Autodesk Fusion 360 part; units mm, degrees
(part 6 of 8)
  spline S141 degree 5 poles (61.3624, 12.8997) (61.363, 12.9) (61.3795, 12.9077) (61.4119, 12.9229) (61.4601, 12.9455) (61.524, 12.976) (61.6029, 13.0142) (61.6817, 13.0528) (61.7603, 13.092) (61.8388, 13.1316) (61.9172, 13.1716) (61.9953, 13.2121) (62.0734, 13.2531) (62.1513, 13.2945) (62.229, 13.3363) (62.3066, 13.3785) (62.3841, 13.4212) (62.4614, 13.4642) (62.5386, 13.5076) (62.6157, 13.5515) (62.6926, 13.5957) (62.7694, 13.6403) (62.846, 13.6853) (62.9225, 13.7307) (62.9989, 13.7764) (63.0751, 13.8226) (63.1512, 13.869) (63.2272, 13.9159) (63.303, 13.963) (63.3787, 14.0106) (63.4542, 14.0585) (63.5297, 14.1067) (63.605, 14.1552) (63.6801, 14.2041) (63.7552, 14.2534) (63.8301, 14.3029) (63.9049, 14.3528) (63.9795, 14.403) (64.054, 14.4536) (64.1284, 14.5044) (64.2027, 14.5556) (64.2768, 14.6071) (64.3508, 14.6589) (64.4247, 14.711) (64.4984, 14.7634) (64.572, 14.8161) (64.6455, 14.8691) (64.7189, 14.9225) (64.7921, 14.9761) (64.8652, 15.03) (64.9382, 15.0842) (65.011, 15.1387) (65.0837, 15.1935) (65.1418, 15.2375) (65.1853, 15.2707) (65.2143, 15.2928) (65.2287, 15.3039) knots 0.270845 0.270845 0.270845 0.270845 0.270845 0.270845 0.271429 0.285714 0.3 0.314286 0.328571 0.342857 0.357143 0.371429 0.385714 0.4 0.414286 0.428571 0.442857 0.457143 0.471429 0.485714 0.5 0.514286 0.528571 0.542857 0.557143 0.571429 0.585714 0.6 0.614286 0.628571 0.642857 0.657143 0.671429 0.685714 0.7 0.714286 0.728571 0.742857 0.757143 0.771429 0.785714 0.8 0.814286 0.828571 0.842857 0.857143 0.871429 0.885714 0.9 0.914286 0.928571 0.942857 0.957143 0.971429 0.985714 1 1 1 1 1 1
  arc A71 (65.2287, 15.3039) -> (64.8693, 16.7623) centre (0, 0) ccw
  spline S142 degree 5 poles (64.8693, 16.7623) (64.8513, 16.7654) (64.8153, 16.7716) (64.7614, 16.7808) (64.6895, 16.7928) (64.5997, 16.8075) (64.5099, 16.8219) (64.4201, 16.836) (64.3303, 16.8497) (64.2405, 16.8632) (64.1508, 16.8763) (64.0611, 16.8891) (63.9714, 16.9016) (63.8818, 16.9137) (63.7921, 16.9255) (63.7025, 16.937) (63.613, 16.9481) (63.5234, 16.9589) (63.4339, 16.9694) (63.3445, 16.9795) (63.255, 16.9893) (63.1656, 16.9987) (63.0763, 17.0078) (62.987, 17.0165) (62.8977, 17.0249) (62.8084, 17.0329) (62.7192, 17.0405) (62.6301, 17.0478) (62.541, 17.0547) (62.4519, 17.0612) (62.3629, 17.0674) (62.2739, 17.0732) (62.185, 17.0786) (62.0961, 17.0836) (62.0073, 17.0882) (61.9185, 17.0925) (61.8298, 17.0963) (61.7411, 17.0997) (61.6525, 17.1027) (61.564, 17.1053) (61.4755, 17.1075) (61.3871, 17.1092) (61.2987, 17.1106) (61.2105, 17.1115) (61.1223, 17.1119) (61.0341, 17.1119) (60.9461, 17.1114) (60.8581, 17.1105) (60.7702, 17.1091) (60.6824, 17.1072) (60.5947, 17.1048) (60.507, 17.1019) (60.4363, 17.0992) (60.3831, 17.0969) (60.3474, 17.0953) (60.3292, 17.0944) (60.3285, 17.0944) knots -1 -1 -1 -1 -1 -1 -0.985714 -0.971429 -0.957143 -0.942857 -0.928571 -0.914286 -0.9 -0.885714 -0.871429 -0.857143 -0.842857 -0.828571 -0.814286 -0.8 -0.785714 -0.771429 -0.757143 -0.742857 -0.728571 -0.714286 -0.7 -0.685714 -0.671429 -0.657143 -0.642857 -0.628571 -0.614286 -0.6 -0.585714 -0.571429 -0.557143 -0.542857 -0.528571 -0.514286 -0.5 -0.485714 -0.471429 -0.457143 -0.442857 -0.428571 -0.414286 -0.4 -0.385714 -0.371429 -0.357143 -0.342857 -0.328571 -0.314286 -0.3 -0.285714 -0.271429 -0.270845 -0.270845 -0.270845 -0.270845 -0.270845 -0.270845
  spline S143 degree 3 poles (60.1267, 17.239) (60.1339, 17.214) (60.1459, 17.1906) (60.1782, 17.1497) (60.1981, 17.1326) (60.2371, 17.1107) (60.2547, 17.1038) (60.2911, 17.0952) (60.3098, 17.0935) (60.3285, 17.0944) knots 0 0 0 0 0.007813 0.007813 0.015626 0.015626 0.021241 0.021241 0.026855 0.026855 0.026855 0.026855
  arc A72 (60.1267, 17.239) -> (59.7414, 18.5303) centre (0, 0) ccw
  spline S144 degree 3 poles (59.8309, 18.7618) (59.8085, 18.7486) (59.7888, 18.7312) (59.7573, 18.6897) (59.7458, 18.6661) (59.7343, 18.6228) (59.7321, 18.6041) (59.7328, 18.5667) (59.7358, 18.5481) (59.7414, 18.5303) knots 0 0 0 0 0.007813 0.007813 0.015626 0.015626 0.021241 0.021241 0.026855 0.026855 0.026855 0.026855
  spline S145 degree 5 poles (59.8309, 18.7618) (59.8315, 18.7622) (59.8472, 18.7715) (59.878, 18.7896) (59.9237, 18.8169) (59.9844, 18.8534) (60.0593, 18.899) (60.134, 18.9451) (60.2085, 18.9916) (60.2828, 19.0386) (60.3569, 19.086) (60.4308, 19.1339) (60.5045, 19.1822) (60.578, 19.2309) (60.6514, 19.28) (60.7246, 19.3295) (60.7975, 19.3794) (60.8704, 19.4297) (60.943, 19.4804) (61.0155, 19.5315) (61.0877, 19.583) (61.1598, 19.6348) (61.2318, 19.687) (61.3035, 19.7395) (61.3751, 19.7924) (61.4466, 19.8457) (61.5178, 19.8993) (61.5889, 19.9532) (61.6598, 20.0075) (61.7306, 20.0621) (61.8012, 20.117) (61.8716, 20.1723) (61.9419, 20.2279) (62.012, 20.2839) (62.0819, 20.3401) (62.1517, 20.3967) (62.2213, 20.4535) (62.2907, 20.5107) (62.36, 20.5682) (62.4292, 20.626) (62.4981, 20.6841) (62.5669, 20.7425) (62.6356, 20.8012) (62.7041, 20.8602) (62.7724, 20.9195) (62.8406, 20.9791) (62.9086, 21.0389) (62.9765, 21.0991) (63.0442, 21.1595) (63.1118, 21.2202) (63.1792, 21.2812) (63.2464, 21.3425) (63.3135, 21.404) (63.3671, 21.4535) (63.4072, 21.4907) (63.4338, 21.5155) (63.4472, 21.528) knots 0.270845 0.270845 0.270845 0.270845 0.270845 0.270845 0.271429 0.285714 0.3 0.314286 0.328571 0.342857 0.357143 0.371429 0.385714 0.4 0.414286 0.428571 0.442857 0.457143 0.471429 0.485714 0.5 0.514286 0.528571 0.542857 0.557143 0.571429 0.585714 0.6 0.614286 0.628571 0.642857 0.657143 0.671429 0.685714 0.7 0.714286 0.728571 0.742857 0.757143 0.771429 0.785714 0.8 0.814286 0.828571 0.842857 0.857143 0.871429 0.885714 0.9 0.914286 0.928571 0.942857 0.957143 0.971429 0.985714 1 1 1 1 1 1
  arc A73 (63.4472, 21.528) -> (62.9487, 22.9449) centre (0, 0) ccw
  spline S146 degree 5 poles (62.9487, 22.9449) (62.9305, 22.9462) (62.8941, 22.9489) (62.8395, 22.9528) (62.7668, 22.9578) (62.676, 22.9638) (62.5852, 22.9695) (62.4944, 22.9748) (62.4037, 22.9798) (62.3131, 22.9846) (62.2225, 22.989) (62.132, 22.993) (62.0415, 22.9968) (61.9511, 23.0002) (61.8608, 23.0033) (61.7705, 23.0061) (61.6803, 23.0085) (61.5901, 23.0106) (61.5, 23.0124) (61.41, 23.0139) (61.32, 23.015) (61.2302, 23.0157) (61.1403, 23.0161) (61.0506, 23.0162) (60.9609, 23.0159) (60.8713, 23.0152) (60.7818, 23.0142) (60.6923, 23.0129) (60.603, 23.0112) (60.5137, 23.0091) (60.4245, 23.0066) (60.3354, 23.0038) (60.2463, 23.0006) (60.1574, 22.997) (60.0685, 22.993) (59.9798, 22.9887) (59.8911, 22.9839) (59.8025, 22.9788) (59.714, 22.9732) (59.6257, 22.9672) (59.5374, 22.9609) (59.4492, 22.9541) (59.3612, 22.9469) (59.2732, 22.9392) (59.1854, 22.9312) (59.0977, 22.9227) (59.0101, 22.9137) (58.9226, 22.9043) (58.8353, 22.8944) (58.748, 22.884) (58.6609, 22.8732) (58.574, 22.8619) (58.5038, 22.8523) (58.4511, 22.8449) (58.4158, 22.8398) (58.3977, 22.8372) (58.397, 22.8371) knots -1 -1 -1 -1 -1 -1 -0.985714 -0.971429 -0.957143 -0.942857 -0.928571 -0.914286 -0.9 -0.885714 -0.871429 -0.857143 -0.842857 -0.828571 -0.814286 -0.8 -0.785714 -0.771429 -0.757143 -0.742857 -0.728571 -0.714286 -0.7 -0.685714 -0.671429 -0.657143 -0.642857 -0.628571 -0.614286 -0.6 -0.585714 -0.571429 -0.557143 -0.542857 -0.528571 -0.514286 -0.5 -0.485714 -0.471429 -0.457143 -0.442857 -0.428571 -0.414286 -0.4 -0.385714 -0.371429 -0.357143 -0.342857 -0.328571 -0.314286 -0.3 -0.285714 -0.271429 -0.270845 -0.270845 -0.270845 -0.270845 -0.270845 -0.270845
  spline S147 degree 3 poles (58.1822, 22.9616) (58.1918, 22.9374) (58.206, 22.9152) (58.242, 22.8777) (58.2636, 22.8626) (58.3045, 22.8445) (58.3226, 22.8394) (58.3597, 22.8343) (58.3785, 22.8344) (58.397, 22.8371) knots 0 0 0 0 0.007813 0.007813 0.015626 0.015626 0.021241 0.021241 0.026855 0.026855 0.026855 0.026855
  arc A74 (58.1822, 22.9616) -> (57.6741, 24.2096) centre (0, 0) ccw
  spline S148 degree 3 poles (57.7408, 24.4488) (57.7198, 24.4335) (57.7019, 24.4142) (57.6746, 24.3698) (57.6653, 24.3452) (57.6581, 24.301) (57.6576, 24.2822) (57.662, 24.2451) (57.6668, 24.2269) (57.6741, 24.2096) knots 0 0 0 0 0.007813 0.007813 0.015626 0.015626 0.021241 0.021241 0.026855 0.026855 0.026855 0.026855
  spline S149 degree 5 poles (57.7408, 24.4488) (57.7414, 24.4492) (57.7561, 24.4599) (57.785, 24.481) (57.8279, 24.5125) (57.8848, 24.5547) (57.9549, 24.6073) (58.0248, 24.6604) (58.0944, 24.7139) (58.1638, 24.7678) (58.233, 24.8222) (58.302, 24.877) (58.3707, 24.9321) (58.4392, 24.9877) (58.5075, 25.0437) (58.5755, 25.1) (58.6433, 25.1568) (58.711, 25.2139) (58.7784, 25.2713) (58.8455, 25.3292) (58.9125, 25.3874) (58.9793, 25.4459) (59.0459, 25.5048) (59.1122, 25.564) (59.1784, 25.6236) (59.2443, 25.6835) (59.3101, 25.7437) (59.3756, 25.8042) (59.441, 25.8651) (59.5061, 25.9263) (59.5711, 25.9878) (59.6359, 26.0496) (59.7004, 26.1117) (59.7648, 26.1742) (59.829, 26.2369) (59.893, 26.2999) (59.9568, 26.3633) (60.0204, 26.4269) (60.0838, 26.4908) (60.147, 26.555) (60.2101, 26.6195) (60.2729, 26.6843) (60.3356, 26.7493) (60.3981, 26.8146) (60.4604, 26.8802) (60.5225, 26.9461) (60.5844, 27.0123) (60.6462, 27.0787) (60.7077, 27.1454) (60.7691, 27.2123) (60.8303, 27.2795) (60.8913, 27.347) (60.9522, 27.4147) (61.0007, 27.4691) (61.037, 27.51) (61.0612, 27.5373) (61.0732, 27.551) knots 0.270845 0.270845 0.270845 0.270845 0.270845 0.270845 0.271429 0.285714 0.3 0.314286 0.328571 0.342857 0.357143 0.371429 0.385714 0.4 0.414286 0.428571 0.442857 0.457143 0.471429 0.485714 0.5 0.514286 0.528571 0.542857 0.557143 0.571429 0.585714 0.6 0.614286 0.628571 0.642857 0.657143 0.671429 0.685714 0.7 0.714286 0.728571 0.742857 0.757143 0.771429 0.785714 0.8 0.814286 0.828571 0.842857 0.857143 0.871429 0.885714 0.9 0.914286 0.928571 0.942857 0.957143 0.971429 0.985714 1 1 1 1 1 1
  arc A75 (61.0732, 27.551) -> (60.4403, 28.9132) centre (0, 0) ccw
  spline S150 degree 5 poles (60.4403, 28.9132) (60.422, 28.9128) (60.3856, 28.9119) (60.3309, 28.9105) (60.258, 28.9085) (60.167, 28.9057) (60.0761, 28.9026) (59.9853, 28.8991) (59.8945, 28.8954) (59.8039, 28.8913) (59.7133, 28.887) (59.6228, 28.8823) (59.5324, 28.8773) (59.4421, 28.872) (59.3519, 28.8664) (59.2617, 28.8604) (59.1717, 28.8541) (59.0818, 28.8475) (58.9919, 28.8406) (58.9022, 28.8333) (58.8125, 28.8257) (58.723, 28.8178) (58.6335, 28.8096) (58.5442, 28.801) (58.455, 28.792) (58.3659, 28.7827) (58.2768, 28.7731) (58.1879, 28.7631) (58.0992, 28.7528) (58.0105, 28.7421) (57.9219, 28.731) (57.8335, 28.7196) (57.7452, 28.7078) (57.657, 28.6957) (57.569, 28.6831) (57.481, 28.6702) (57.3932, 28.6569) (57.3056, 28.6433) (57.218, 28.6292) (57.1307, 28.6147) (57.0434, 28.5999) (56.9563, 28.5846) (56.8694, 28.5689) (56.7826, 28.5528) (56.6959, 28.5363) (56.6094, 28.5194) (56.5231, 28.502) (56.4369, 28.4842) (56.351, 28.4659) (56.2651, 28.4472) (56.1795, 28.428) (56.0941, 28.4084) (56.0252, 28.3921) (55.9734, 28.3796) (55.9387, 28.3711) (55.921, 28.3668) (55.9203, 28.3666) knots -1 -1 -1 -1 -1 -1 -0.985714 -0.971429 -0.957143 -0.942857 -0.928571 -0.914286 -0.9 -0.885714 -0.871429 -0.857143 -0.842857 -0.828571 -0.814286 -0.8 -0.785714 -0.771429 -0.757143 -0.742857 -0.728571 -0.714286 -0.7 -0.685714 -0.671429 -0.657143 -0.642857 -0.628571 -0.614286 -0.6 -0.585714 -0.571429 -0.557143 -0.542857 -0.528571 -0.514286 -0.5 -0.485714 -0.471429 -0.457143 -0.442857 -0.428571 -0.414286 -0.4 -0.385714 -0.371429 -0.357143 -0.342857 -0.328571 -0.314286 -0.3 -0.285714 -0.271429 -0.270845 -0.270845 -0.270845 -0.270845 -0.270845 -0.270845
  spline S151 degree 3 poles (55.6945, 28.4698) (55.7063, 28.4466) (55.7226, 28.426) (55.7621, 28.3921) (55.785, 28.3791) (55.8275, 28.3651) (55.846, 28.3617) (55.8834, 28.3602) (55.9021, 28.3621) (55.9203, 28.3666) knots 0 0 0 0 0.007813 0.007813 0.015626 0.015626 0.021241 0.021241 0.026855 0.026855 0.026855 0.026855
  arc A76 (55.6945, 28.4698) -> (55.0682, 29.663) centre (0, 0) ccw
  spline S152 degree 3 poles (55.1116, 29.9074) (55.0921, 29.8902) (55.0762, 29.8692) (55.0533, 29.8225) (55.0465, 29.7971) (55.0435, 29.7524) (55.0449, 29.7337) (55.0528, 29.6971) (55.0594, 29.6794) (55.0682, 29.663) knots 0 0 0 0 0.007813 0.007813 0.015626 0.015626 0.021241 0.021241 0.026855 0.026855 0.026855 0.026855
  spline S153 degree 5 poles (55.1116, 29.9074) (55.1122, 29.9079) (55.1258, 29.92) (55.1525, 29.9437) (55.1921, 29.9793) (55.2447, 30.0267) (55.3094, 30.0859) (55.3738, 30.1455) (55.438, 30.2054) (55.5019, 30.2658) (55.5655, 30.3266) (55.6288, 30.3878) (55.6919, 30.4493) (55.7547, 30.5113) (55.8173, 30.5736) (55.8795, 30.6362) (55.9416, 30.6992) (56.0034, 30.7626) (56.0649, 30.8263) (56.1262, 30.8903) (56.1873, 30.9547) (56.2481, 31.0194) (56.3087, 31.0845) (56.369, 31.1498) (56.4291, 31.2155) (56.4889, 31.2815) (56.5486, 31.3477) (56.608, 31.4143) (56.6671, 31.4812) (56.7261, 31.5484) (56.7848, 31.6159) (56.8433, 31.6837) (56.9016, 31.7518) (56.9596, 31.8201) (57.0174, 31.8888) (57.0751, 31.9577) (57.1324, 32.0269) (57.1896, 32.0963) (57.2466, 32.1661) (57.3033, 32.2361) (57.3598, 32.3063) (57.4161, 32.3769) (57.4722, 32.4477) (57.5281, 32.5187) (57.5838, 32.59) (57.6393, 32.6616) (57.6945, 32.7334) (57.7496, 32.8055) (57.8044, 32.8778) (57.859, 32.9503) (57.9135, 33.0231) (57.9677, 33.0962) (58.0217, 33.1695) (58.0648, 33.2283) (58.097, 33.2725) (58.1184, 33.302) (58.1291, 33.3168) knots 0.270845 0.270845 0.270845 0.270845 0.270845 0.270845 0.271429 0.285714 0.3 0.314286 0.328571 0.342857 0.357143 0.371429 0.385714 0.4 0.414286 0.428571 0.442857 0.457143 0.471429 0.485714 0.5 0.514286 0.528571 0.542857 0.557143 0.571429 0.585714 0.6 0.614286 0.628571 0.642857 0.657143 0.671429 0.685714 0.7 0.714286 0.728571 0.742857 0.757143 0.771429 0.785714 0.8 0.814286 0.828571 0.842857 0.857143 0.871429 0.885714 0.9 0.914286 0.928571 0.942857 0.957143 0.971429 0.985714 1 1 1 1 1 1
  arc A77 (58.1291, 33.3168) -> (57.3676, 34.6115) centre (0, 0) ccw
  spline S154 degree 5 poles (57.3676, 34.6115) (57.3495, 34.6094) (57.3133, 34.605) (57.259, 34.5983) (57.1866, 34.5893) (57.0963, 34.5777) (57.0062, 34.5658) (56.9161, 34.5536) (56.8261, 34.5411) (56.7363, 34.5284) (56.6465, 34.5153) (56.5569, 34.5019) (56.4674, 34.4882) (56.378, 34.4742) (56.2888, 34.4599) (56.1996, 34.4453) (56.1106, 34.4303) (56.0217, 34.4151) (55.933, 34.3995) (55.8444, 34.3836) (55.7559, 34.3674) (55.6675, 34.3509) (55.5793, 34.334) (55.4912, 34.3168) (55.4033, 34.2993) (55.3154, 34.2815) (55.2278, 34.2633) (55.1403, 34.2448) (55.0529, 34.2259) (54.9657, 34.2067) (54.8786, 34.1872) (54.7917, 34.1673) (54.7049, 34.147) (54.6183, 34.1264) (54.5319, 34.1054) (54.4456, 34.0841) (54.3595, 34.0624) (54.2736, 34.0403) (54.1878, 34.0179) (54.1022, 33.9951) (54.0168, 33.9718) (53.9316, 33.9482) (53.8466, 33.9242) (53.7617, 33.8999) (53.6771, 33.8751) (53.5926, 33.8499) (53.5084, 33.8242) (53.4244, 33.7982) (53.3405, 33.7717) (53.2569, 33.7448) (53.1736, 33.7174) (53.0904, 33.6896) (53.0234, 33.6667) (52.9731, 33.6493) (52.9393, 33.6376) (52.9222, 33.6315) (52.9215, 33.6313) knots -1 -1 -1 -1 -1 -1 -0.985714 -0.971429 -0.957143 -0.942857 -0.928571 -0.914286 -0.9 -0.885714 -0.871429 -0.857143 -0.842857 -0.828571 -0.814286 -0.8 -0.785714 -0.771429 -0.757143 -0.742857 -0.728571 -0.714286 -0.7 -0.685714 -0.671429 -0.657143 -0.642857 -0.628571 -0.614286 -0.6 -0.585714 -0.571429 -0.557143 -0.542857 -0.528571 -0.514286 -0.5 -0.485714 -0.471429 -0.457143 -0.442857 -0.428571 -0.414286 -0.4 -0.385714 -0.371429 -0.357143 -0.342857 -0.328571 -0.314286 -0.3 -0.285714 -0.271429 -0.270845 -0.270845 -0.270845 -0.270845 -0.270845 -0.270845
  spline S155 degree 3 poles (52.6867, 33.7122) (52.7008, 33.6902) (52.719, 33.6713) (52.7616, 33.6413) (52.7856, 33.6307) (52.8293, 33.6208) (52.848, 33.6192) (52.8854, 33.6214) (52.9038, 33.6251) (52.9215, 33.6313) knots 0 0 0 0 0.007813 0.007813 0.015626 0.015626 0.021241 0.021241 0.026855 0.026855 0.026855 0.026855
  arc A78 (52.6867, 33.7122) -> (51.9483, 34.8393) centre (0, 0) ccw
  spline S156 degree 3 poles (51.9679, 35.0869) (51.9501, 35.0678) (51.9363, 35.0454) (51.918, 34.9967) (51.9137, 34.9707) (51.915, 34.926) (51.9182, 34.9074) (51.9297, 34.8718) (51.9379, 34.8549) (51.9483, 34.8393) knots 0 0 0 0 0.007813 0.007813 0.015626 0.015626 0.021241 0.021241 0.026855 0.026855 0.026855 0.026855
  spline S157 degree 5 poles (51.9679, 35.0869) (51.9683, 35.0874) (51.9807, 35.1007) (52.005, 35.1269) (52.0411, 35.1661) (52.0888, 35.2184) (52.1475, 35.2836) (52.2059, 35.3491) (52.2639, 35.415) (52.3217, 35.4812) (52.3791, 35.5479) (52.4363, 35.6149) (52.4931, 35.6822) (52.5497, 35.7499) (52.6059, 35.818) (52.6619, 35.8864) (52.7175, 35.9551) (52.7729, 36.0241) (52.828, 36.0934) (52.8829, 36.1631) (52.9374, 36.2331) (52.9917, 36.3033) (53.0457, 36.3739) (53.0994, 36.4448) (53.1529, 36.5159) (53.2061, 36.5874) (53.2591, 36.6591) (53.3118, 36.7311) (53.3642, 36.8034) (53.4164, 36.876) (53.4683, 36.9489) (53.52, 37.022) (53.5715, 37.0953) (53.6226, 37.169) (53.6736, 37.2429) (53.7242, 37.317) (53.7747, 37.3914) (53.8249, 37.4661) (53.8748, 37.541) (53.9246, 37.6161) (53.974, 37.6915) (54.0233, 37.7672) (54.0723, 37.8431) (54.1211, 37.9192) (54.1696, 37.9955) (54.2179, 38.0721) (54.266, 38.1489) (54.3138, 38.226) (54.3614, 38.3032) (54.4088, 38.3807) (54.4559, 38.4584) (54.5028, 38.5364) (54.5495, 38.6145) (54.5867, 38.6772) (54.6145, 38.7244) (54.6329, 38.7558) (54.6422, 38.7716) knots 0.270845 0.270845 0.270845 0.270845 0.270845 0.270845 0.271429 0.285714 0.3 0.314286 0.328571 0.342857 0.357143 0.371429 0.385714 0.4 0.414286 0.428571 0.442857 0.457143 0.471429 0.485714 0.5 0.514286 0.528571 0.542857 0.557143 0.571429 0.585714 0.6 0.614286 0.628571 0.642857 0.657143 0.671429 0.685714 0.7 0.714286 0.728571 0.742857 0.757143 0.771429 0.785714 0.8 0.814286 0.828571 0.842857 0.857143 0.871429 0.885714 0.9 0.914286 0.928571 0.942857 0.957143 0.971429 0.985714 1 1 1 1 1 1
  arc A79 (54.6422, 38.7716) -> (53.7593, 39.9867) centre (0, 0) ccw
  spline S158 degree 5 poles (53.7593, 39.9867) (53.7415, 39.9828) (53.7058, 39.975) (53.6524, 39.9631) (53.5813, 39.9471) (53.4926, 39.9269) (53.404, 39.9063) (53.3155, 39.8855) (53.2271, 39.8644) (53.1389, 39.843) (53.0509, 39.8213) (52.963, 39.7993) (52.8752, 39.7771) (52.7876, 39.7545) (52.7001, 39.7317) (52.6128, 39.7085) (52.5257, 39.685) (52.4387, 39.6613) (52.3518, 39.6372) (52.2652, 39.6129) (52.1787, 39.5882) (52.0923, 39.5632) (52.0061, 39.5379) (51.9201, 39.5123) (51.8342, 39.4864) (51.7486, 39.4602) (51.6631, 39.4336) (51.5778, 39.4067) (51.4926, 39.3795) (51.4076, 39.352) (51.3229, 39.3241) (51.2383, 39.2959) (51.1539, 39.2674) (51.0697, 39.2385) (50.9857, 39.2093) (50.9019, 39.1797) (50.8182, 39.1498) (50.7348, 39.1196) (50.6517, 39.0889) (50.5687, 39.058) (50.4859, 39.0266) (50.4034, 38.9949) (50.321, 38.9628) (50.2389, 38.9304) (50.1571, 38.8975) (50.0755, 38.8643) (49.9941, 38.8306) (49.913, 38.7966) (49.8321, 38.7621) (49.7515, 38.7273) (49.6711, 38.692) (49.591, 38.6563) (49.5265, 38.6271) (49.4781, 38.6049) (49.4457, 38.5899) (49.4292, 38.5822) (49.4285, 38.5819) knots -1 -1 -1 -1 -1 -1 -0.985714 -0.971429 -0.957143 -0.942857 -0.928571 -0.914286 -0.9 -0.885714 -0.871429 -0.857143 -0.842857 -0.828571 -0.814286 -0.8 -0.785714 -0.771429 -0.757143 -0.742857 -0.728571 -0.714286 -0.7 -0.685714 -0.671429 -0.657143 -0.642857 -0.628571 -0.614286 -0.6 -0.585714 -0.571429 -0.557143 -0.542857 -0.528571 -0.514286 -0.5 -0.485714 -0.471429 -0.457143 -0.442857 -0.428571 -0.414286 -0.4 -0.385714 -0.371429 -0.357143 -0.342857 -0.328571 -0.314286 -0.3 -0.285714 -0.271429 -0.270845 -0.270845 -0.270845 -0.270845 -0.270845 -0.270845
  spline S159 degree 3 poles (49.1871, 38.6398) (49.2032, 38.6193) (49.2231, 38.6022) (49.2684, 38.5765) (49.2934, 38.5682) (49.3378, 38.5626) (49.3566, 38.5629) (49.3936, 38.5686) (49.4116, 38.5741) (49.4285, 38.5819) knots 0 0 0 0 0.007813 0.007813 0.015626 0.015626 0.021241 0.021241 0.026855 0.026855 0.026855 0.026855
  arc A80 (49.1871, 38.6398) -> (48.3433, 39.6904) centre (0, 0) ccw
  spline S160 degree 3 poles (48.3389, 39.9387) (48.3231, 39.918) (48.3115, 39.8944) (48.298, 39.8441) (48.2962, 39.8179) (48.3018, 39.7735) (48.3068, 39.7553) (48.3216, 39.7209) (48.3314, 39.7049) (48.3433, 39.6904) knots 0 0 0 0 0.007813 0.007813 0.015626 0.015626 0.021241 0.021241 0.026855 0.026855 0.026855 0.026855
  spline S161 degree 5 poles (48.3389, 39.9387) (48.3393, 39.9392) (48.3504, 39.9537) (48.372, 39.9822) (48.4041, 40.0246) (48.4465, 40.0813) (48.4987, 40.1518) (48.5505, 40.2226) (48.6019, 40.2938) (48.653, 40.3654) (48.7038, 40.4372) (48.7542, 40.5094) (48.8042, 40.582) (48.854, 40.6548) (48.9034, 40.728) (48.9525, 40.8014) (49.0013, 40.8752) (49.0497, 40.9492) (49.0979, 41.0236) (49.1457, 41.0982) (49.1933, 41.1731) (49.2405, 41.2483) (49.2875, 41.3238) (49.3341, 41.3995) (49.3805, 41.4755) (49.4266, 41.5517) (49.4723, 41.6282) (49.5178, 41.705) (49.5631, 41.782) (49.608, 41.8593) (49.6527, 41.9368) (49.697, 42.0146) (49.7411, 42.0926) (49.785, 42.1708) (49.8285, 42.2493) (49.8718, 42.3279) (49.9149, 42.4069) (49.9576, 42.486) (50.0001, 42.5654) (50.0423, 42.645) (50.0843, 42.7248) (50.126, 42.8049) (50.1675, 42.8851) (50.2087, 42.9656) (50.2496, 43.0463) (50.2903, 43.1272) (50.3307, 43.2082) (50.3709, 43.2895) (50.4108, 43.371) (50.4505, 43.4528) (50.4899, 43.5347) (50.5291, 43.6168) (50.568, 43.699) (50.599, 43.765) (50.6221, 43.8146) (50.6374, 43.8477) (50.6451, 43.8643) knots 0.270845 0.270845 0.270845 0.270845 0.270845 0.270845 0.271429 0.285714 0.3 0.314286 0.328571 0.342857 0.357143 0.371429 0.385714 0.4 0.414286 0.428571 0.442857 0.457143 0.471429 0.485714 0.5 0.514286 0.528571 0.542857 0.557143 0.571429 0.585714 0.6 0.614286 0.628571 0.642857 0.657143 0.671429 0.685714 0.7 0.714286 0.728571 0.742857 0.757143 0.771429 0.785714 0.8 0.814286 0.828571 0.842857 0.857143 0.871429 0.885714 0.9 0.914286 0.928571 0.942857 0.957143 0.971429 0.985714 1 1 1 1 1 1
  arc A81 (50.6451, 43.8643) -> (49.6491, 44.9886) centre (0, 0) ccw
  spline S162 degree 5 poles (49.6491, 44.9886) (49.6317, 44.983) (49.597, 44.9717) (49.545, 44.9548) (49.4757, 44.932) (49.3893, 44.9033) (49.3031, 44.8743) (49.2171, 44.845) (49.1312, 44.8155) (49.0455, 44.7857) (48.9599, 44.7556) (48.8745, 44.7252) (48.7893, 44.6946) (48.7043, 44.6637) (48.6195, 44.6325) (48.5348, 44.601) (48.4503, 44.5692) (48.366, 44.5372) (48.2819, 44.5049) (48.198, 44.4722) (48.1143, 44.4393) (48.0307, 44.4061) (47.9474, 44.3726) (47.8642, 44.3389) (47.7813, 44.3048) (47.6985, 44.2704) (47.616, 44.2357) (47.5337, 44.2007) (47.4516, 44.1654) (47.3696, 44.1298) (47.288, 44.0939) (47.2065, 44.0577) (47.1252, 44.0211) (47.0442, 43.9843) (46.9634, 43.9471) (46.8828, 43.9096) (46.8025, 43.8717) (46.7224, 43.8336) (46.6426, 43.7951) (46.563, 43.7562) (46.4836, 43.717) (46.4045, 43.6775) (46.3257, 43.6376) (46.2471, 43.5974) (46.1688, 43.5568) (46.0907, 43.5158) (46.013, 43.4745) (45.9355, 43.4328) (45.8584, 43.3907) (45.7815, 43.3482) (45.7049, 43.3053) (45.6287, 43.262) (45.5673, 43.2267) (45.5212, 43.2) (45.4904, 43.1819) (45.4747, 43.1727) (45.4741, 43.1724) knots -1 -1 -1 -1 -1 -1 -0.985714 -0.971429 -0.957143 -0.942857 -0.928571 -0.914286 -0.9 -0.885714 -0.871429 -0.857143 -0.842857 -0.828571 -0.814286 -0.8 -0.785714 -0.771429 -0.757143 -0.742857 -0.728571 -0.714286 -0.7 -0.685714 -0.671429 -0.657143 -0.642857 -0.628571 -0.614286 -0.6 -0.585714 -0.571429 -0.557143 -0.542857 -0.528571 -0.514286 -0.5 -0.485714 -0.471429 -0.457143 -0.442857 -0.428571 -0.414286 -0.4 -0.385714 -0.371429 -0.357143 -0.342857 -0.328571 -0.314286 -0.3 -0.285714 -0.271429 -0.270845 -0.270845 -0.270845 -0.270845 -0.270845 -0.270845
  spline S163 degree 3 poles (45.2282, 43.2067) (45.2462, 43.1878) (45.2677, 43.1727) (45.3152, 43.1515) (45.3409, 43.1457) (45.3856, 43.1443) (45.4043, 43.1464) (45.4406, 43.1557) (45.458, 43.1629) (45.4741, 43.1724) knots 0 0 0 0 0.007813 0.007813 0.015626 0.015626 0.021241 0.021241 0.026855 0.026855 0.026855 0.026855
  arc A82 (45.2282, 43.2067) -> (44.2869, 44.1709) centre (0, 0) ccw
  spline S164 degree 3 poles (44.2586, 44.4176) (44.2449, 44.3955) (44.2356, 44.3709) (44.227, 44.3195) (44.2277, 44.2932) (44.2377, 44.2496) (44.2443, 44.232) (44.2624, 44.1992) (44.2737, 44.1842) (44.2869, 44.1709) knots 0 0 0 0 0.007813 0.007813 0.015626 0.015626 0.021241 0.021241 0.026855 0.026855 0.026855 0.026855
  spline S165 degree 5 poles (44.2586, 44.4176) (44.259, 44.4182) (44.2686, 44.4337) (44.2873, 44.4641) (44.3152, 44.5095) (44.352, 44.57) (44.3971, 44.6452) (44.4418, 44.7207) (44.4861, 44.7965) (44.5301, 44.8726) (44.5736, 44.9491) (44.6168, 45.0258) (44.6597, 45.1028) (44.7021, 45.1801) (44.7443, 45.2577) (44.786, 45.3355) (44.8275, 45.4137) (44.8686, 45.492) (44.9093, 45.5707) (44.9498, 45.6496) (44.9898, 45.7287) (45.0296, 45.8081) (45.0691, 45.8878) (45.1082, 45.9676) (45.147, 46.0478) (45.1855, 46.1281) (45.2237, 46.2087) (45.2616, 46.2895) (45.2991, 46.3705) (45.3364, 46.4517) (45.3734, 46.5332) (45.41, 46.6149) (45.4464, 46.6968) (45.4825, 46.7789) (45.5183, 46.8612) (45.5538, 46.9437) (45.589, 47.0264) (45.6239, 47.1093) (45.6585, 47.1924) (45.6929, 47.2757) (45.727, 47.3592) (45.7608, 47.4429) (45.7943, 47.5268) (45.8275, 47.6108) (45.8605, 47.6951) (45.8931, 47.7795) (45.9256, 47.8641) (45.9577, 47.9489) (45.9896, 48.0339) (46.0212, 48.1191) (46.0525, 48.2044) (46.0836, 48.2899) (46.1144, 48.3756) (46.1388, 48.4442) (46.157, 48.4958) (46.1691, 48.5302) (46.1751, 48.5475) knots 0.270845 0.270845 0.270845 0.270845 0.270845 0.270845 0.271429 0.285714 0.3 0.314286 0.328571 0.342857 0.357143 0.371429 0.385714 0.4 0.414286 0.428571 0.442857 0.457143 0.471429 0.485714 0.5 0.514286 0.528571 0.542857 0.557143 0.571429 0.585714 0.6 0.614286 0.628571 0.642857 0.657143 0.671429 0.685714 0.7 0.714286 0.728571 0.742857 0.757143 0.771429 0.785714 0.8 0.814286 0.828571 0.842857 0.857143 0.871429 0.885714 0.9 0.914286 0.928571 0.942857 0.957143 0.971429 0.985714 1 1 1 1 1 1
  arc A83 (46.1751, 48.5475) -> (45.0752, 49.5704) centre (0, 0) ccw
  spline S166 degree 5 poles (45.0752, 49.5704) (45.0585, 49.5631) (45.0251, 49.5486) (44.9749, 49.5267) (44.9082, 49.4973) (44.825, 49.4604) (44.742, 49.4232) (44.6591, 49.3858) (44.5765, 49.3481) (44.4941, 49.3102) (44.4118, 49.272) (44.3298, 49.2335) (44.2479, 49.1948) (44.1663, 49.1558) (44.0848, 49.1166) (44.0036, 49.0771) (43.9226, 49.0373) (43.8418, 48.9973) (43.7612, 48.957) (43.6808, 48.9164) (43.6006, 48.8756) (43.5207, 48.8345) (43.441, 48.7931) (43.3615, 48.7514) (43.2822, 48.7095) (43.2032, 48.6673) (43.1244, 48.6248) (43.0458, 48.582) (42.9675, 48.539) (42.8894, 48.4956) (42.8115, 48.452) (42.7339, 48.4081) (42.6566, 48.3639) (42.5795, 48.3194) (42.5027, 48.2745) (42.4261, 48.2294) (42.3498, 48.184) (42.2737, 48.1383) (42.198, 48.0923) (42.1225, 48.0459) (42.0473, 47.9993) (41.9724, 47.9523) (41.8978, 47.905) (41.8234, 47.8573) (41.7494, 47.8094) (41.6757, 47.7611) (41.6023, 47.7124) (41.5292, 47.6634) (41.4565, 47.6141) (41.3841, 47.5644) (41.312, 47.5143) (41.2403, 47.4639) (41.1826, 47.4228) (41.1393, 47.3918) (41.1104, 47.3708) (41.0956, 47.3601) (41.0951, 47.3597) knots -1 -1 -1 -1 -1 -1 -0.985714 -0.971429 -0.957143 -0.942857 -0.928571 -0.914286 -0.9 -0.885714 -0.871429 -0.857143 -0.842857 -0.828571 -0.814286 -0.8 -0.785714 -0.771429 -0.757143 -0.742857 -0.728571 -0.714286 -0.7 -0.685714 -0.671429 -0.657143 -0.642857 -0.628571 -0.614286 -0.6 -0.585714 -0.571429 -0.557143 -0.542857 -0.528571 -0.514286 -0.5 -0.485714 -0.471429 -0.457143 -0.442857 -0.428571 -0.414286 -0.4 -0.385714 -0.371429 -0.357143 -0.342857 -0.328571 -0.314286 -0.3 -0.285714 -0.271429 -0.270845 -0.270845 -0.270845 -0.270845 -0.270845 -0.270845
  spline S167 degree 3 poles (40.847, 47.3701) (40.8667, 47.3531) (40.8896, 47.3401) (40.939, 47.3236) (40.965, 47.3203) (41.0097, 47.3233) (41.0281, 47.3271) (41.0633, 47.3399) (41.0799, 47.3487) (41.0951, 47.3597) knots 0 0 0 0 0.007813 0.007813 0.015626 0.015626 0.021241 0.021241 0.026855 0.026855 0.026855 0.026855
  arc A84 (40.847, 47.3701) -> (39.8171, 48.239) centre (0, 0) ccw
  spline S168 degree 3 poles (39.765, 48.4818) (39.7535, 48.4585) (39.7467, 48.4331) (39.7431, 48.3811) (39.7463, 48.355) (39.7604, 48.3126) (39.7688, 48.2957) (39.7899, 48.2648) (39.8026, 48.2509) (39.8171, 48.239) knots 0 0 0 0 0.007813 0.007813 0.015626 0.015626 0.021241 0.021241 0.026855 0.026855 0.026855 0.026855
  spline S169 degree 5 poles (39.765, 48.4818) (39.7654, 48.4825) (39.7734, 48.4988) (39.7892, 48.5308) (39.8125, 48.5787) (39.8433, 48.6425) (39.8809, 48.7217) (39.9181, 48.8011) (39.955, 48.8809) (39.9913, 48.9609) (40.0273, 49.0412) (40.0629, 49.1217) (40.0981, 49.2025) (40.133, 49.2836) (40.1674, 49.3649) (40.2015, 49.4464) (40.2352, 49.5281) (40.2685, 49.6101) (40.3015, 49.6923) (40.3341, 49.7748) (40.3664, 49.8574) (40.3983, 49.9403) (40.4299, 50.0233) (40.4611, 50.1066) (40.492, 50.1901) (40.5226, 50.2738) (40.5528, 50.3577) (40.5827, 50.4417) (40.6123, 50.526) (40.6415, 50.6105) (40.6705, 50.6951) (40.6991, 50.78) (40.7274, 50.865) (40.7554, 50.9502) (40.783, 51.0355) (40.8104, 51.1211) (40.8375, 51.2068) (40.8642, 51.2927) (40.8907, 51.3788) (40.9168, 51.465) (40.9427, 51.5514) (40.9682, 51.638) (40.9935, 51.7247) (41.0185, 51.8116) (41.0431, 51.8986) (41.0675, 51.9858) (41.0916, 52.0732) (41.1154, 52.1607) (41.1389, 52.2483) (41.1622, 52.3361) (41.1851, 52.4241) (41.2078, 52.5122) (41.2302, 52.6004) (41.2479, 52.6711) (41.261, 52.7242) (41.2697, 52.7596) (41.2741, 52.7774) knots 0.270845 0.270845 0.270845 0.270845 0.270845 0.270845 0.271429 0.285714 0.3 0.314286 0.328571 0.342857 0.357143 0.371429 0.385714 0.4 0.414286 0.428571 0.442857 0.457143 0.471429 0.485714 0.5 0.514286 0.528571 0.542857 0.557143 0.571429 0.585714 0.6 0.614286 0.628571 0.642857 0.657143 0.671429 0.685714 0.7 0.714286 0.728571 0.742857 0.757143 0.771429 0.785714 0.8 0.814286 0.828571 0.842857 0.857143 0.871429 0.885714 0.9 0.914286 0.928571 0.942857 0.957143 0.971429 0.985714 1 1 1 1 1 1
  arc A85 (41.2741, 52.7774) -> (40.0806, 53.6893) centre (0, 0) ccw
  spline S170 degree 5 poles (40.0806, 53.6893) (40.0646, 53.6805) (40.0327, 53.6628) (39.985, 53.6362) (39.9214, 53.6005) (39.8421, 53.5557) (39.7631, 53.5107) (39.6842, 53.4655) (39.6056, 53.42) (39.5272, 53.3742) (39.449, 53.3283) (39.3711, 53.2821) (39.2934, 53.2357) (39.2159, 53.189) (39.1386, 53.1421) (39.0616, 53.0949) (38.9847, 53.0475) (38.9082, 52.9999) (38.8318, 52.952) (38.7558, 52.9039) (38.6799, 52.8555) (38.6043, 52.8068) (38.5289, 52.758) (38.4538, 52.7088) (38.379, 52.6594) (38.3044, 52.6098) (38.2301, 52.5599) (38.156, 52.5098) (38.0822, 52.4593) (38.0086, 52.4087) (37.9354, 52.3577) (37.8624, 52.3065) (37.7897, 52.255) (37.7172, 52.2033) (37.6451, 52.1513) (37.5732, 52.099) (37.5016, 52.0464) (37.4304, 51.9936) (37.3594, 51.9404) (37.2888, 51.887) (37.2184, 51.8333) (37.1484, 51.7793) (37.0787, 51.725) (37.0093, 51.6705) (36.9402, 51.6156) (36.8715, 51.5604) (36.8032, 51.5049) (36.7352, 51.4491) (36.6675, 51.3929) (36.6002, 51.3365) (36.5333, 51.2797) (36.4668, 51.2226) (36.4134, 51.1761) (36.3733, 51.141) (36.3465, 51.1174) (36.3329, 51.1053) (36.3323, 51.1049) knots -1 -1 -1 -1 -1 -1 -0.985714 -0.971429 -0.957143 -0.942857 -0.928571 -0.914286 -0.9 -0.885714 -0.871429 -0.857143 -0.842857 -0.828571 -0.814286 -0.8 -0.785714 -0.771429 -0.757143 -0.742857 -0.728571 -0.714286 -0.7 -0.685714 -0.671429 -0.657143 -0.642857 -0.628571 -0.614286 -0.6 -0.585714 -0.571429 -0.557143 -0.542857 -0.528571 -0.514286 -0.5 -0.485714 -0.471429 -0.457143 -0.442857 -0.428571 -0.414286 -0.4 -0.385714 -0.371429 -0.357143 -0.342857 -0.328571 -0.314286 -0.3 -0.285714 -0.271429 -0.270845 -0.270845 -0.270845 -0.270845 -0.270845 -0.270845
  spline S171 degree 3 poles (36.0844, 51.0913) (36.1057, 51.0762) (36.1297, 51.0655) (36.1805, 51.0539) (36.2067, 51.0531) (36.2509, 51.0604) (36.2688, 51.066) (36.3026, 51.0821) (36.3183, 51.0924) (36.3323, 51.1049) knots 0 0 0 0 0.007813 0.007813 0.015626 0.015626 0.021241 0.021241 0.026855 0.026855 0.026855 0.026855
  arc A86 (36.0844, 51.0913) -> (34.9754, 51.8567) centre (0, 0) ccw
  spline S172 degree 3 poles (34.9002, 52.0934) (34.891, 52.069) (34.8866, 52.0431) (34.8881, 51.991) (34.8939, 51.9654) (34.912, 51.9245) (34.9219, 51.9085) (34.946, 51.8798) (34.9599, 51.8672) (34.9754, 51.8567) knots 0 0 0 0 0.007813 0.007813 0.015626 0.015626 0.021241 0.021241 0.026855 0.026855 0.026855 0.026855
  spline S173 degree 5 poles (34.9002, 52.0934) (34.9005, 52.094) (34.9069, 52.1111) (34.9195, 52.1445) (34.9382, 52.1944) (34.9626, 52.2608) (34.9924, 52.3433) (35.0218, 52.426) (35.0507, 52.5089) (35.0792, 52.5921) (35.1073, 52.6754) (35.135, 52.759) (35.1622, 52.8429) (35.189, 52.9269) (35.2155, 53.0111) (35.2415, 53.0955) (35.2672, 53.1802) (35.2924, 53.265) (35.3173, 53.35) (35.3418, 53.4352) (35.366, 53.5206) (35.3898, 53.6061) (35.4132, 53.6919) (35.4362, 53.7778) (35.4589, 53.8638) (35.4813, 53.9501) (35.5033, 54.0365) (35.5249, 54.1231) (35.5462, 54.2098) (35.5672, 54.2967) (35.5878, 54.3837) (35.6081, 54.4709) (35.6281, 54.5583) (35.6477, 54.6458) (35.667, 54.7334) (35.686, 54.8212) (35.7046, 54.9092) (35.723, 54.9972) (35.741, 55.0854) (35.7587, 55.1738) (35.7761, 55.2623) (35.7932, 55.3509) (35.81, 55.4397) (35.8264, 55.5285) (35.8426, 55.6176) (35.8584, 55.7067) (35.874, 55.796) (35.8892, 55.8854) (35.9042, 55.9749) (35.9189, 56.0645) (35.9332, 56.1543) (35.9473, 56.2441) (35.961, 56.3341) (35.9718, 56.4062) (35.9798, 56.4603) (35.985, 56.4965) (35.9876, 56.5145) knots 0.270845 0.270845 0.270845 0.270845 0.270845 0.270845 0.271429 0.285714 0.3 0.314286 0.328571 0.342857 0.357143 0.371429 0.385714 0.4 0.414286 0.428571 0.442857 0.457143 0.471429 0.485714 0.5 0.514286 0.528571 0.542857 0.557143 0.571429 0.585714 0.6 0.614286 0.628571 0.642857 0.657143 0.671429 0.685714 0.7 0.714286 0.728571 0.742857 0.757143 0.771429 0.785714 0.8 0.814286 0.828571 0.842857 0.857143 0.871429 0.885714 0.9 0.914286 0.928571 0.942857 0.957143 0.971429 0.985714 1 1 1 1 1 1
  arc A87 (35.9876, 56.5145) -> (34.7117, 57.307) centre (0, 0) ccw
  spline S174 degree 5 poles (34.7117, 57.307) (34.6967, 57.2967) (34.6666, 57.276) (34.6217, 57.2449) (34.5618, 57.2033) (34.4872, 57.151) (34.4129, 57.0986) (34.3388, 57.0459) (34.265, 56.9931) (34.1913, 56.94) (34.118, 56.8867) (34.0448, 56.8332) (33.9719, 56.7795) (33.8993, 56.7256) (33.8269, 56.6714) (33.7548, 56.617) (33.6829, 56.5624) (33.6113, 56.5076) (33.54, 56.4526) (33.4689, 56.3973) (33.398, 56.3419) (33.3275, 56.2862) (33.2572, 56.2302) (33.1872, 56.1741) (33.1175, 56.1177) (33.048, 56.0611) (32.9788, 56.0043) (32.9099, 55.9472) (32.8413, 55.8899) (32.773, 55.8324) (32.705, 55.7746) (32.6373, 55.7166) (32.5699, 55.6583) (32.5028, 55.5998) (32.436, 55.5411) (32.3695, 55.4821) (32.3034, 55.4229) (32.2375, 55.3634) (32.172, 55.3037) (32.1069, 55.2437) (32.042, 55.1834) (31.9775, 55.1229) (31.9134, 55.0622) (31.8496, 55.0012) (31.7862, 54.9399) (31.7231, 54.8783) (31.6604, 54.8165) (31.5981, 54.7543) (31.5362, 54.6919) (31.4747, 54.6292) (31.4136, 54.5663) (31.3529, 54.503) (31.3042, 54.4516) (31.2677, 54.4128) (31.2433, 54.3867) (31.2309, 54.3734) (31.2304, 54.3729) knots -1 -1 -1 -1 -1 -1 -0.985714 -0.971429 -0.957143 -0.942857 -0.928571 -0.914286 -0.9 -0.885714 -0.871429 -0.857143 -0.842857 -0.828571 -0.814286 -0.8 -0.785714 -0.771429 -0.757143 -0.742857 -0.728571 -0.714286 -0.7 -0.685714 -0.671429 -0.657143 -0.642857 -0.628571 -0.614286 -0.6 -0.585714 -0.571429 -0.557143 -0.542857 -0.528571 -0.514286 -0.5 -0.485714 -0.471429 -0.457143 -0.442857 -0.428571 -0.414286 -0.4 -0.385714 -0.371429 -0.357143 -0.342857 -0.328571 -0.314286 -0.3 -0.285714 -0.271429 -0.270845 -0.270845 -0.270845 -0.270845 -0.270845 -0.270845
  spline S175 degree 3 poles (30.9849, 54.3354) (31.0076, 54.3225) (31.0325, 54.3141) (31.0842, 54.3074) (31.1104, 54.3092) (31.1536, 54.3207) (31.171, 54.328) (31.203, 54.3473) (31.2177, 54.3592) (31.2304, 54.3729) knots 0 0 0 0 0.007813 0.007813 0.015626 0.015626 0.021241 0.021241 0.026855 0.026855 0.026855 0.026855
  arc A88 (30.9849, 54.3354) -> (29.8073, 54.9903) centre (0, 0) ccw
  spline S176 degree 3 poles (29.7096, 55.2185) (29.7027, 55.1934) (29.7009, 55.1672) (29.7073, 55.1155) (29.7156, 55.0905) (29.7376, 55.0515) (29.749, 55.0366) (29.7757, 55.0104) (29.7908, 54.9992) (29.8073, 54.9903) knots 0 0 0 0 0.007813 0.007813 0.015626 0.015626 0.021241 0.021241 0.026855 0.026855 0.026855 0.026855
  spline S177 degree 5 poles (29.7096, 55.2185) (29.7098, 55.2192) (29.7145, 55.2368) (29.7238, 55.2713) (29.7376, 55.3227) (29.7555, 55.3912) (29.7772, 55.4762) (29.7985, 55.5613) (29.8193, 55.6467) (29.8396, 55.7322) (29.8595, 55.8179) (29.879, 55.9038) (29.898, 55.9898) (29.9166, 56.076) (29.9348, 56.1624) (29.9525, 56.249) (29.9699, 56.3357) (29.9869, 56.4225) (30.0034, 56.5096) (30.0196, 56.5967) (30.0354, 56.684) (30.0508, 56.7715) (30.0658, 56.8591) (30.0805, 56.9468) (30.0948, 57.0347) (30.1087, 57.1227) (30.1222, 57.2108) (30.1354, 57.299) (30.1483, 57.3874) (30.1607, 57.4759) (30.1729, 57.5646) (30.1847, 57.6533) (30.1961, 57.7422) (30.2072, 57.8312) (30.218, 57.9203) (30.2284, 58.0095) (30.2385, 58.0988) (30.2482, 58.1882) (30.2576, 58.2778) (30.2667, 58.3674) (30.2755, 58.4572) (30.284, 58.547) (30.2921, 58.637) (30.2999, 58.7271) (30.3074, 58.8172) (30.3146, 58.9075) (30.3214, 58.9978) (30.328, 59.0883) (30.3342, 59.1788) (30.3402, 59.2695) (30.3458, 59.3602) (30.3511, 59.451) (30.3561, 59.5419) (30.3599, 59.6147) (30.3626, 59.6693) (30.3643, 59.7058) (30.3652, 59.724) knots 0.270845 0.270845 0.270845 0.270845 0.270845 0.270845 0.271429 0.285714 0.3 0.314286 0.328571 0.342857 0.357143 0.371429 0.385714 0.4 0.414286 0.428571 0.442857 0.457143 0.471429 0.485714 0.5 0.514286 0.528571 0.542857 0.557143 0.571429 0.585714 0.6 0.614286 0.628571 0.642857 0.657143 0.671429 0.685714 0.7 0.714286 0.728571 0.742857 0.757143 0.771429 0.785714 0.8 0.814286 0.828571 0.842857 0.857143 0.871429 0.885714 0.9 0.914286 0.928571 0.942857 0.957143 0.971429 0.985714 1 1 1 1 1 1
  arc A89 (30.3652, 59.724) -> (29.0187, 60.3897) centre (0, 0) ccw
  spline S178 degree 5 poles (29.0187, 60.3897) (29.0048, 60.3779) (28.9769, 60.3544) (28.9351, 60.3191) (28.8796, 60.2719) (28.8104, 60.2127) (28.7414, 60.1534) (28.6728, 60.0938) (28.6044, 60.0341) (28.5362, 59.9741) (28.4683, 59.914) (28.4007, 59.8537) (28.3333, 59.7932) (28.2663, 59.7325) (28.1994, 59.6716) (28.1329, 59.6105) (28.0666, 59.5493) (28.0006, 59.4878) (27.9349, 59.4261) (27.8695, 59.3643) (27.8044, 59.3022) (27.7395, 59.24) (27.6749, 59.1775) (27.6107, 59.1149) (27.5467, 59.052) (27.483, 58.989) (27.4197, 58.9257) (27.3566, 58.8623) (27.2939, 58.7986) (27.2314, 58.7348) (27.1693, 58.6707) (27.1075, 58.6064) (27.046, 58.5419) (26.9849, 58.4772) (26.9241, 58.4123) (26.8636, 58.3472) (26.8035, 58.2819) (26.7437, 58.2163) (26.6843, 58.1505) (26.6252, 58.0845) (26.5665, 58.0183) (26.5081, 57.9519) (26.4501, 57.8852) (26.3925, 57.8183) (26.3353, 57.7512) (26.2785, 57.6838) (26.2221, 57.6162) (26.166, 57.5484) (26.1105, 57.4803) (26.0553, 57.412) (26.0005, 57.3434) (25.9462, 57.2745) (25.9027, 57.2187) (25.8701, 57.1766) (25.8484, 57.1482) (25.8373, 57.1338) (25.8369, 57.1332) knots -1 -1 -1 -1 -1 -1 -0.985714 -0.971429 -0.957143 -0.942857 -0.928571 -0.914286 -0.9 -0.885714 -0.871429 -0.857143 -0.842857 -0.828571 -0.814286 -0.8 -0.785714 -0.771429 -0.757143 -0.742857 -0.728571 -0.714286 -0.7 -0.685714 -0.671429 -0.657143 -0.642857 -0.628571 -0.614286 -0.6 -0.585714 -0.571429 -0.557143 -0.542857 -0.528571 -0.514286 -0.5 -0.485714 -0.471429 -0.457143 -0.442857 -0.428571 -0.414286 -0.4 -0.385714 -0.371429 -0.357143 -0.342857 -0.328571 -0.314286 -0.3 -0.285714 -0.271429 -0.270845 -0.270845 -0.270845 -0.270845 -0.270845 -0.270845
  spline S179 degree 3 poles (25.5962, 57.0722) (25.6199, 57.0616) (25.6456, 57.0556) (25.6976, 57.054) (25.7236, 57.0582) (25.7655, 57.0739) (25.782, 57.0829) (25.8121, 57.1051) (25.8255, 57.1183) (25.8369, 57.1332) knots 0 0 0 0 0.007813 0.007813 0.015626 0.015626 0.021241 0.021241 0.026855 0.026855 0.026855 0.026855
  arc A90 (25.5962, 57.0722) -> (24.3608, 57.6104) centre (0, 0) ccw
  spline S180 degree 3 poles (24.2415, 57.8281) (24.2372, 57.8025) (24.2378, 57.7762) (24.2492, 57.7254) (24.2599, 57.7013) (24.2855, 57.6646) (24.2983, 57.6509) (24.3274, 57.6273) (24.3436, 57.6177) (24.3608, 57.6104) knots 0 0 0 0 0.007813 0.007813 0.015626 0.015626 0.021241 0.021241 0.026855 0.026855 0.026855 0.026855
  spline S181 degree 5 poles (24.2415, 57.8281) (24.2416, 57.8288) (24.2447, 57.8468) (24.2506, 57.882) (24.2593, 57.9346) (24.2706, 58.0045) (24.284, 58.0911) (24.2969, 58.1779) (24.3094, 58.2649) (24.3214, 58.3519) (24.3329, 58.4392) (24.344, 58.5265) (24.3546, 58.614) (24.3648, 58.7016) (24.3746, 58.7894) (24.3839, 58.8772) (24.3928, 58.9652) (24.4013, 59.0533) (24.4094, 59.1415) (24.4171, 59.2298) (24.4244, 59.3182) (24.4313, 59.4068) (24.4378, 59.4954) (24.4439, 59.5841) (24.4496, 59.673) (24.455, 59.7619) (24.46, 59.8509) (24.4646, 59.94) (24.4688, 60.0292) (24.4727, 60.1185) (24.4762, 60.2079) (24.4794, 60.2974) (24.4822, 60.387) (24.4847, 60.4766) (24.4868, 60.5663) (24.4885, 60.6561) (24.49, 60.746) (24.491, 60.836) (24.4918, 60.926) (24.4922, 61.0161) (24.4922, 61.1063) (24.492, 61.1966) (24.4914, 61.2869) (24.4905, 61.3773) (24.4892, 61.4677) (24.4877, 61.5583) (24.4858, 61.6489) (24.4836, 61.7395) (24.481, 61.8302) (24.4782, 61.921) (24.475, 62.0119) (24.4716, 62.1028) (24.4678, 62.1937) (24.4645, 62.2665) (24.4619, 62.3212) (24.4602, 62.3576) (24.4592, 62.3758) knots 0.270845 0.270845 0.270845 0.270845 0.270845 0.270845 0.271429 0.285714 0.3 0.314286 0.328571 0.342857 0.357143 0.371429 0.385714 0.4 0.414286 0.428571 0.442857 0.457143 0.471429 0.485714 0.5 0.514286 0.528571 0.542857 0.557143 0.571429 0.585714 0.6 0.614286 0.628571 0.642857 0.657143 0.671429 0.685714 0.7 0.714286 0.728571 0.742857 0.757143 0.771429 0.785714 0.8 0.814286 0.828571 0.842857 0.857143 0.871429 0.885714 0.9 0.914286 0.928571 0.942857 0.957143 0.971429 0.985714 1 1 1 1 1 1
  arc A91 (24.4592, 62.3758) -> (23.0548, 62.9085) centre (0, 0) ccw
  spline S182 degree 5 poles (23.0548, 62.9085) (23.0421, 62.8954) (23.0166, 62.8693) (22.9784, 62.8302) (22.9277, 62.7778) (22.8645, 62.7122) (22.8016, 62.6465) (22.739, 62.5806) (22.6767, 62.5145) (22.6147, 62.4483) (22.5529, 62.3819) (22.4914, 62.3153) (22.4302, 62.2486) (22.3693, 62.1817) (22.3086, 62.1147) (22.2483, 62.0475) (22.1883, 61.9801) (22.1285, 61.9125) (22.0691, 61.8448) (22.0099, 61.7769) (21.9511, 61.7089) (21.8925, 61.6407) (21.8343, 61.5723) (21.7764, 61.5037) (21.7188, 61.435) (21.6615, 61.3661) (21.6045, 61.297) (21.5479, 61.2278) (21.4916, 61.1584) (21.4356, 61.0888) (21.3799, 61.019) (21.3246, 60.9491) (21.2697, 60.879) (21.2151, 60.8087) (21.1608, 60.7382) (21.1069, 60.6675) (21.0533, 60.5967) (21.0002, 60.5257) (20.9474, 60.4545) (20.8949, 60.3831) (20.8429, 60.3115) (20.7912, 60.2397) (20.7399, 60.1678) (20.6891, 60.0957) (20.6386, 60.0233) (20.5885, 59.9508) (20.5389, 59.878) (20.4897, 59.8051) (20.4409, 59.732) (20.3926, 59.6586) (20.3447, 59.5851) (20.2973, 59.5113) (20.2594, 59.4516) (20.231, 59.4065) (20.2121, 59.3762) (20.2025, 59.3607) (20.2021, 59.3601) knots -1 -1 -1 -1 -1 -1 -0.985714 -0.971429 -0.957143 -0.942857 -0.928571 -0.914286 -0.9 -0.885714 -0.871429 -0.857143 -0.842857 -0.828571 -0.814286 -0.8 -0.785714 -0.771429 -0.757143 -0.742857 -0.728571 -0.714286 -0.7 -0.685714 -0.671429 -0.657143 -0.642857 -0.628571 -0.614286 -0.6 -0.585714 -0.571429 -0.557143 -0.542857 -0.528571 -0.514286 -0.5 -0.485714 -0.471429 -0.457143 -0.442857 -0.428571 -0.414286 -0.4 -0.385714 -0.371429 -0.357143 -0.342857 -0.328571 -0.314286 -0.3 -0.285714 -0.271429 -0.270845 -0.270845 -0.270845 -0.270845 -0.270845 -0.270845
  spline S183 degree 3 poles (19.9684, 59.2762) (19.9931, 59.2679) (20.0192, 59.2644) (20.0711, 59.2678) (20.0966, 59.2745) (20.1368, 59.2942) (20.1524, 59.3047) (20.1802, 59.3298) (20.1922, 59.3442) (20.2021, 59.3601) knots 0 0 0 0 0.007813 0.007813 0.015626 0.015626 0.021241 0.021241 0.026855 0.026855 0.026855 0.026855
  arc A92 (19.9684, 59.2762) -> (18.6869, 59.6926) centre (0, 0) ccw
  spline S184 degree 3 poles (18.5471, 59.8978) (18.5453, 59.8718) (18.5485, 59.8458) (18.5647, 59.7963) (18.5776, 59.7734) (18.6067, 59.7393) (18.6208, 59.7269) (18.652, 59.7062) (18.669, 59.6982) (18.6869, 59.6926) knots 0 0 0 0 0.007813 0.007813 0.015626 0.015626 0.021241 0.021241 0.026855 0.026855 0.026855 0.026855
  spline S185 degree 5 poles (18.5471, 59.8978) (18.5472, 59.8985) (18.5485, 59.9167) (18.551, 59.9523) (18.5546, 60.0055) (18.559, 60.0761) (18.564, 60.1637) (18.5685, 60.2513) (18.5725, 60.339) (18.5761, 60.4269) (18.5791, 60.5148) (18.5817, 60.6028) (18.5839, 60.6909) (18.5855, 60.7791) (18.5868, 60.8674) (18.5876, 60.9557) (18.588, 61.0442) (18.5879, 61.1327) (18.5875, 61.2212) (18.5866, 61.3099) (18.5853, 61.3986) (18.5836, 61.4874) (18.5816, 61.5762) (18.5791, 61.6651) (18.5762, 61.7541) (18.573, 61.8431) (18.5693, 61.9322) (18.5653, 62.0214) (18.5609, 62.1106) (18.5562, 62.1998) (18.5511, 62.2892) (18.5456, 62.3785) (18.5397, 62.4679) (18.5335, 62.5574) (18.527, 62.6469) (18.5201, 62.7365) (18.5128, 62.8261) (18.5052, 62.9157) (18.4972, 63.0054) (18.4889, 63.0951) (18.4803, 63.1849) (18.4713, 63.2747) (18.462, 63.3645) (18.4524, 63.4544) (18.4424, 63.5443) (18.4321, 63.6343) (18.4215, 63.7243) (18.4105, 63.8143) (18.3993, 63.9043) (18.3877, 63.9944) (18.3758, 64.0845) (18.3636, 64.1747) (18.351, 64.2649) (18.3407, 64.337) (18.3329, 64.3912) (18.3276, 64.4273) (18.3249, 64.4453) knots 0.270845 0.270845 0.270845 0.270845 0.270845 0.270845 0.271429 0.285714 0.3 0.314286 0.328571 0.342857 0.357143 0.371429 0.385714 0.4 0.414286 0.428571 0.442857 0.457143 0.471429 0.485714 0.5 0.514286 0.528571 0.542857 0.557143 0.571429 0.585714 0.6 0.614286 0.628571 0.642857 0.657143 0.671429 0.685714 0.7 0.714286 0.728571 0.742857 0.757143 0.771429 0.785714 0.8 0.814286 0.828571 0.842857 0.857143 0.871429 0.885714 0.9 0.914286 0.928571 0.942857 0.957143 0.971429 0.985714 1 1 1 1 1 1
  arc A93 (18.3249, 64.4453) -> (16.8756, 64.8399) centre (0, 0) ccw
  spline S186 degree 5 poles (16.8756, 64.8399) (16.8642, 64.8257) (16.8413, 64.7973) (16.8071, 64.7546) (16.7617, 64.6976) (16.7052, 64.6262) (16.6489, 64.5547) (16.593, 64.4831) (16.5373, 64.4113) (16.482, 64.3394) (16.4269, 64.2673) (16.3721, 64.1952) (16.3176, 64.1228) (16.2634, 64.0504) (16.2096, 63.9778) (16.156, 63.9051) (16.1027, 63.8322) (16.0498, 63.7592) (15.9972, 63.6861) (15.9448, 63.6128) (15.8928, 63.5394) (15.8411, 63.4658) (15.7898, 63.3922) (15.7387, 63.3183) (15.688, 63.2444) (15.6377, 63.1703) (15.5876, 63.096) (15.5379, 63.0216) (15.4886, 62.9471) (15.4396, 62.8724) (15.3909, 62.7976) (15.3427, 62.7227) (15.2947, 62.6476) (15.2471, 62.5723) (15.1999, 62.497) (15.1531, 62.4214) (15.1066, 62.3458) (15.0606, 62.2699) (15.0149, 62.194) (14.9696, 62.1178) (14.9247, 62.0416) (14.8802, 61.9652) (14.8361, 61.8886) (14.7924, 61.8119) (14.7491, 61.735) (14.7063, 61.658) (14.6639, 61.5808) (14.622, 61.5035) (14.5805, 61.426) (14.5395, 61.3483) (14.4989, 61.2705) (14.4589, 61.1925) (14.4269, 61.1293) (14.403, 61.0817) (14.3871, 61.0497) (14.379, 61.0334) (14.3787, 61.0328) knots -1 -1 -1 -1 -1 -1 -0.985714 -0.971429 -0.957143 -0.942857 -0.928571 -0.914286 -0.9 -0.885714 -0.871429 -0.857143 -0.842857 -0.828571 -0.814286 -0.8 -0.785714 -0.771429 -0.757143 -0.742857 -0.728571 -0.714286 -0.7 -0.685714 -0.671429 -0.657143 -0.642857 -0.628571 -0.614286 -0.6 -0.585714 -0.571429 -0.557143 -0.542857 -0.528571 -0.514286 -0.5 -0.485714 -0.471429 -0.457143 -0.442857 -0.428571 -0.414286 -0.4 -0.385714 -0.371429 -0.357143 -0.342857 -0.328571 -0.314286 -0.3 -0.285714 -0.271429 -0.270845 -0.270845 -0.270845 -0.270845 -0.270845 -0.270845
  spline S187 degree 3 poles (14.1542, 60.9267) (14.1796, 60.9208) (14.2059, 60.9199) (14.2573, 60.9283) (14.2819, 60.9374) (14.3201, 60.9608) (14.3346, 60.9728) (14.3598, 61.0005) (14.3704, 61.016) (14.3787, 61.0328) knots 0 0 0 0 0.007813 0.007813 0.015626 0.015626 0.021241 0.021241 0.026855 0.026855 0.026855 0.026855
  arc A94 (14.1542, 60.9267) -> (12.8385, 61.2175) centre (0, 0) ccw
  spline S188 degree 3 poles (12.6796, 61.4083) (12.6802, 61.3822) (12.6859, 61.3566) (12.7069, 61.3089) (12.7219, 61.2873) (12.7542, 61.2562) (12.7694, 61.2452) (12.8025, 61.2277) (12.8201, 61.2213) (12.8385, 61.2175) knots 0 0 0 0 0.007813 0.007813 0.015626 0.015626 0.021241 0.021241 0.026855 0.026855 0.026855 0.026855